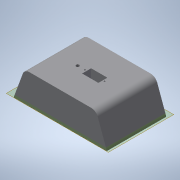
# Autodesk Inventor part: cover-new
Saved by Autodesk Inventor 2020 (Build 240168000, 168)
## iProperties
Created: 2020-08-26
Part Number: cover-new
Material: Ogólny
Document SubType Name: Modeling
Designer: blep
Density: 1 g/cm^3
Appearance: Domyślna
Author: blep
Autodesk Inventor part; units mm, degrees
ref_plane "YZ Plane" through (0, 0, 0) normal (1, 0, 0) x (0, 1, 0)
ref_plane "XZ Plane" through (0, 0, 0) normal (0, 1, 0) x (-1, 0, 0)
ref_plane "XY Plane" through (0, 0, 0) normal (0, 0, 1) x (1, 0, 0)
sketch "Szkic1" plane through (0, 0, 0) normal (0, 0, 1) x (1, 0, 0)
  line L0 (-135, 20) -> (0, 20) projected
  line L1 (-135, 7) -> (-135, 20) projected
  line L2 (0, 7) -> (0, 20) projected
  line L3 (-135, 20) -> (-119.3493, 63)
  line L4 (-119.3493, 63) -> (-15.6507, 63)
  line L5 (-15.6507, 63) -> (0, 20)
  line L6 (-135, 20) -> (-131.8075, 20)
  line L7 (-131.8075, 20) -> (-117.2487, 60)
  line L8 (-117.2487, 60) -> (-17.7513, 60)
  line L9 (-17.7513, 60) -> (-3.1925, 20)
  line L10 (-3.1925, 20) -> (0, 20)
  point P0 (0, 0)
  point P1 (-3.1925, 20)
  dimension "d0" = 3
  dimension "d1" = 3
  dimension "d2" = 3
  dimension "d3" = 40
  dimension "d4" = 70
  dimension "d5" = 70
  constraints: 16 end point, 4 horizontal, 3 parallel
  measures "d0" distance between parallel lines of L3 L7
  measures "d1" distance between parallel lines of L4 L8
  measures "d2" distance between parallel lines of L5 L9
  measures "d3" distance between parallel lines of L8 L0
  measures "d4" angle of L0 L7
  measures "d5" angle of L0 L9
ref_plane "Płaszczyzna konstrukcyjna1" through (-135, -3, -86) normal (0, 0, -1) x (0, 1, 0)
extrude "Wyciągnięcie proste1" add sketch "Szkic1" against normal up to surface (86 mm away) contours L3 L4 L5 L0 L9 L8 L7
sketch "Szkic2" plane through (0, 0, 0) normal (0, 0, 1) x (1, 0, 0)
  line L0 (-131.8075, 20) -> (-117.2487, 60) projected
  line L1 (-117.2487, 60) -> (-17.7513, 60) projected
  line L2 (-17.7513, 60) -> (-3.1925, 20) projected
  line L3 (-131.8075, 20) -> (-3.1925, 20)
  point P0 (0, 0)
  constraints: 2 end point, 1 horizontal
ref_plane "Płaszczyzna konstrukcyjna2" through (-135, -3, -86) normal (0, 0, -1) x (0, 1, 0)
extrude "Wyciągnięcie proste2" add sketch "Szkic2" against normal up to surface (86 mm away)
extrude "Wyciągnięcie proste3" cut sketch "Szkic2" against normal blind 83
extrude "Wyciągnięcie proste4" add sketch "Szkic2" against normal blind 3
sketch "Szkic3" plane through (-135, 20, -86) normal (-0.9396926, 0.3420201, 0) x (0, 0, 1)
  circle A0 centre (63.5, 28.7596) radius 7.75
  line L0 (15, 36.7596) -> (42, 36.7596)
  line L1 (42, 36.7596) -> (42, 16.7596)
  line L2 (42, 16.7596) -> (15, 16.7596)
  line L3 (15, 16.7596) -> (15, 36.7596)
  line L4 (22, 16.7596) -> (35, 16.7596)
  line L5 (35, 16.7596) -> (35, 13.7596)
  line L6 (35, 13.7596) -> (22, 13.7596)
  line L7 (22, 13.7596) -> (22, 16.7596)
  line L8 (86, 45.7596) -> (0, 45.7596) projected
  line L9 (0, 45.7596) -> (0, 0) projected
  line L10 (86, 0) -> (0, 0) projected
  line L11 (86, 45.7596) -> (86, 0) projected
  line L12 (86, 45.7596) -> (0, 45.7596) projected
  line L13 (86, 0) -> (0, 0) construction
  line L14 (42, 36.7596) -> (63.5, 28.7596) construction
  line L15 (15, 20.7596) -> (42, 20.7596) construction
  line L16 (42, 20.7596) -> (63.5, 28.7596) construction
  point P0 (86, 27.3789)
  dimension "d14" = 27
  dimension "d15" = 20
  dimension "d16" = 3
  dimension "d17" = 7
  dimension "d18" = 7
  dimension "d19" = 15.5
  dimension "d20" = 17
  dimension "d23" = 15
  dimension "d36" = 4
  dimension "d42" = 22.5
  constraints: 22 end point, 4 parallel, 3 horizontal, 2 perpendicular, 2 point on line, 1 centre point, 1 collinear, 1 equal length
  measures "d14" distance of L1.end L2.end
  measures "d15" distance of L0.end L1.end
  measures "d16" distance of L4.end L5.end
  measures "d17" distance between parallel lines of L3 L7
  measures "d18" distance between parallel lines of L1 L5
  measures "d19" diameter of A0
  measures "d20" distance from line of L8 L14.end
  measures "d23" distance between parallel lines of L9 L3
  measures "d36" distance between parallel lines of L4 L15
  measures "d42" distance from line of L11 L14.end
extrude "Wyciągnięcie proste5" cut sketch "Szkic3" against normal up to surface (3 mm away) contours A0 | L0 L1 L2 L3 | L2 L5 L6 L7
sketch "Szkic4" plane through (-135, 20, -86) normal (-0.9396926, 0.3420201, 0) x (0, 0, 1)
  line L0 (15, 20.7596) -> (42, 20.7596)
  line L1 (42, 20.7596) -> (42, 16.7596)
  line L2 (42, 16.7596) -> (15, 16.7596)
  line L3 (15, 16.7596) -> (15, 20.7596)
  line L4 (22, 16.7596) -> (35, 16.7596)
  line L5 (35, 16.7596) -> (35, 13.7596)
  line L6 (35, 13.7596) -> (22, 13.7596)
  line L7 (22, 13.7596) -> (22, 16.7596)
  line L8 (35, 13.7596) -> (22, 13.7596) projected
  line L9 (22, 13.7596) -> (22, 16.7596) projected
  line L10 (35, 16.7596) -> (35, 13.7596) projected
  line L11 (42, 36.7596) -> (42, 16.7596) projected
  line L12 (15, 16.7596) -> (15, 36.7596) projected
  line L13 (22, 16.7596) -> (15, 16.7596) projected
  point P0 (86, 27.3789)
  dimension "d26" = 4
  constraints: 16 end point, 7 collinear, 4 parallel, 2 horizontal, 2 perpendicular
  measures "d26" distance between parallel lines of L2 L0
extrude "Wyciągnięcie proste6" add sketch "Szkic4" against normal blind 1
fillet "Zaokrąglenie1" radius 10 2 edges at (-119.3493, 63, -43) (-15.6507, 63, -43)
sketch "Szkic5" plane through (0, 0, 0) normal (0, 0, 1) x (1, 0, 0)
  line L0 (-121.7441, 56.4202) -> (-135, 20) projected
  line L1 (-135, 7) -> (-135, 20) projected
  line L2 (-135, 20) -> (0, 20) projected
  arc A0 (-112.3472, 63) -> (-121.7441, 56.4202) centre (-112.3472, 53) ccw projected
  line L3 (-133.7939, 23.3139) -> (-121.7441, 56.4202)
  line L4 (-135, 16.4735) -> (-135, 7)
  arc A1 (-133.7939, 23.3139) -> (-135, 16.4735) centre (-115, 16.4735) ccw
  line L5 (0, 7) -> (0, 20) projected
  line L6 (0, 20) -> (-13.2559, 56.4202) projected
  line L7 (0, 16.4735) -> (0, 7)
  line L8 (0, 20) -> (-13.2559, 56.4202) projected
  line L9 (-1.2061, 23.3139) -> (-13.2559, 56.4202)
  arc A2 (0, 16.4735) -> (-1.2061, 23.3139) centre (-20, 16.4735) ccw
  line L10 (0, 7) -> (-135, 7)
  line L11 (-121.7441, 56.4202) -> (-119.3493, 63)
  line L12 (-119.3493, 63) -> (-15.6507, 63)
  line L13 (-15.6507, 63) -> (-13.2559, 56.4202)
  line L14 (-22.6528, 63) -> (-112.3472, 63) projected
  point P0 (0, 0)
  dimension "d30" = 20
  dimension "d31" = 20
  constraints: 16 end point, 6 collinear, 5 tangent, 4 point on circle, 4 point on line, 2 centre point, 1 perpendicular, 1 vertical
  measures "d30" radius of A1
  measures "d31" radius of A2
extrude "Wyciągnięcie proste7" cut sketch "Szkic5" against normal through all contours A0 L12 L13 L6 A2 L2 A1 L0 | L2 A2 L5 L10 L1 A1 keep common part
sketch "Szkic6" plane through (-134.6866, 20, 0) normal (0, -1, 0) x (1, 0, 0)
  arc A0 (2.8554, -3) -> (2.6866, -3.1688) centre (5.6866, -6) ccw projected
  line L0 (2.8554, -3) -> (2.6866, -3) projected
  line L1 (2.6866, -3) -> (2.6866, -3.1688) projected
  circle A1 centre (128.6866, -6) radius 2.125 projected
  circle A2 centre (128.6866, -80) radius 2.125 projected
  circle A3 centre (5.6866, -80) radius 2.125 projected
  line L2 (2.6866, -82.8312) -> (2.6866, -83) projected
  line L3 (2.6866, -83) -> (2.8554, -83) projected
  arc A4 (2.6866, -82.8312) -> (2.8554, -83) centre (5.6866, -80) ccw projected
  circle A5 centre (5.6866, -6) radius 2.125 projected
  line L4 (2.6866, -8.8312) -> (2.6866, -77.1688) projected
  arc A6 (8.5178, -83) -> (2.6866, -77.1688) centre (5.6866, -80) ccw projected
  line L5 (8.5178, -83) -> (71.1366, -83) projected
  line L6 (71.1366, -83) -> (71.1366, -75.35) projected
  line L7 (71.1366, -75.35) -> (79.1366, -75.35) projected
  line L8 (79.1366, -75.35) -> (79.1366, -83) projected
  line L9 (79.1366, -83) -> (120.2366, -83) projected
  line L10 (120.2366, -83) -> (120.2366, -75.35) projected
  line L11 (120.2366, -75.35) -> (131.6866, -75.35) projected
  line L12 (131.6866, -75.35) -> (131.6866, -10.65) projected
  line L13 (131.6866, -10.65) -> (120.2366, -10.65) projected
  line L14 (120.2366, -10.65) -> (120.2366, -3) projected
  line L15 (120.2366, -3) -> (79.1366, -3) projected
  line L16 (79.1366, -3) -> (79.1366, -10.65) projected
  line L17 (79.1366, -10.65) -> (71.1366, -10.65) projected
  line L18 (71.1366, -10.65) -> (71.1366, -3) projected
  line L19 (71.1366, -3) -> (8.5178, -3) projected
  arc A7 (2.6866, -8.8312) -> (8.5178, -3) centre (5.6866, -6) ccw projected
  line L20 (0, 0) -> (0, -86) projected
  line L21 (0, 0) -> (134.3733, 0) projected
  line L22 (134.3733, -86) -> (134.3733, 0) projected
  line L23 (134.3733, -86) -> (0, -86) projected
  circle A8 centre (5.6866, -6) radius 4.125
  circle A9 centre (5.6866, -6) radius 2.125
  circle A10 centre (128.6866, -6) radius 2.125
  circle A11 centre (128.6866, -6) radius 4.125
  circle A12 centre (128.6866, -80) radius 2.125
  circle A13 centre (128.6866, -80) radius 4.125
  circle A14 centre (5.6866, -80) radius 2.125
  circle A15 centre (5.6866, -80) radius 4.125
  point P0 (134.6866, 0)
  point P1 (2.6866, -3.1688)
  point P2 (2.8554, -3)
  point P3 (8.5178, -83)
  point P4 (2.6866, -77.1688)
  constraints: 8 centre point, 8 coincident, 8 equal radius
extrude "Wyciągnięcie proste8" add sketch "Szkic6" against normal through all contours A8 A7 A0 | A6 A15 A4 | A11 | A13
ref_plane "Płaszczyzna konstrukcyjna3" through (-134.6866, 24, 0) normal (0, -1, 0) x (1, 0, 0)
sketch "Szkic11" plane through (-134.6866, 24, 0) normal (0, -1, 0) x (1, 0, 0)
  arc A0 (8.5178, -83) -> (2.8792, -76.9778) centre (5.6866, -80) ccw projected
  arc A1 (125.8554, -3) -> (131.4941, -9.0222) centre (128.6866, -6) ccw projected
  arc A2 (131.4941, -76.9778) -> (125.8554, -83) centre (128.6866, -80) ccw projected
  arc A3 (2.8792, -9.0222) -> (8.5178, -3) centre (5.6866, -6) ccw projected
  circle A4 centre (5.6866, -80) radius 4.125
  circle A5 centre (5.6866, -6) radius 4.125
  circle A6 centre (128.6866, -6) radius 4.125
  circle A7 centre (128.6866, -80) radius 4.125
  circle A8 centre (128.6866, -80) radius 2.125 projected
  circle A9 centre (128.6866, -6) radius 2.125 projected
  circle A10 centre (5.6866, -80) radius 2.125 projected
  circle A11 centre (5.6866, -6) radius 2.125 projected
  point P0 (8.5178, -3)
  point P1 (131.4941, -9.0222)
  point P2 (125.8554, -3)
  point P3 (125.8554, -83)
  point P4 (2.8792, -76.9778)
  constraints: 4 centre point, 4 coincident, 4 concentric
extrude "Wyciągnięcie proste9" cut sketch "Szkic11" along normal blind 3 contours A4 A0 | A6 A1 | A7 A2 | A5 A3 | A8 | A9 | A10 | A11
sketch "Szkic12" plane through (-134.6866, 20, 0) normal (0, -1, 0) x (1, 0, 0)
  circle A0 centre (5.6866, -80) radius 2.125 projected
  circle A1 centre (128.6866, -6) radius 2.125 projected
  line L0 (134.3733, 0) -> (134.3733, -86) projected
  line L1 (0, 0) -> (134.3733, 0) projected
  line L2 (0, -86) -> (0, 0) projected
  line L3 (0, -86) -> (134.3733, -86) projected
  circle A2 centre (5.6866, -6) radius 2.125 projected
  circle A3 centre (128.6866, -80) radius 2.125 projected
  arc A4 (131.4941, -76.9778) -> (125.8554, -83) centre (128.6866, -80) ccw projected
  line L4 (125.8554, -83) -> (8.5178, -83) projected
  arc A5 (8.5178, -83) -> (2.8792, -76.9778) centre (5.6866, -80) ccw projected
  line L5 (2.8792, -76.9778) -> (2.8792, -9.0222) projected
  arc A6 (2.8792, -9.0222) -> (8.5178, -3) centre (5.6866, -6) ccw projected
  line L6 (125.8554, -3) -> (8.5178, -3) projected
  arc A7 (125.8554, -3) -> (131.4941, -9.0222) centre (128.6866, -6) ccw projected
  line L7 (131.4941, -9.0222) -> (131.4941, -76.9778) projected
  point P0 (134.6866, 0)
extrude "Wyciągnięcie proste10" cut sketch "Szkic12" against normal blind 8 contours A0 | A1 | A2 | A3
sketch "Szkic13" plane through (-112.3472, 63, -86) normal (0, 1, 0) x (1, 0, 0)
  line L0 (68.5, -49.5) -> (35, -49.5)
  line L1 (35, -49.5) -> (35, -36.5)
  line L2 (35, -36.5) -> (68.5, -36.5)
  line L3 (68.5, -36.5) -> (68.5, -49.5)
  line L4 (89.6944, -86) -> (0, -86) projected
  line L5 (89.6944, 0) -> (0, 0) projected
  line L6 (89.6944, 0) -> (89.6944, -86) projected
  line L7 (0, -86) -> (0, 0) projected
  line L8 (99.0913, -86) -> (89.6944, -86) construction
  line L9 (68.5, -49.5) -> (89.6944, -86) construction
  line L10 (68.5, -36.5) -> (89.6944, 0) construction
  line L11 (63.5, -49.5) -> (63.5, -36.5)
  line L12 (40, -49.5) -> (40, -36.5)
  line L13 (68.5, -49.5) -> (66, -43) construction
  line L14 (66, -43) -> (63.5, -36.5) construction
  line L15 (68.5, -36.5) -> (66, -43) construction
  line L16 (40, -49.5) -> (37.5, -43) construction
  line L17 (37.5, -43) -> (35, -36.5) construction
  line L18 (37.5, -43) -> (40, -36.5) construction
  circle A0 centre (27, -43) radius 2.25
  line L19 (0, -86) -> (27, -43) construction
  line L20 (0, 0) -> (27, -43) construction
  circle A1 centre (57, -43) radius 1.5065 construction
  point P0 (112.3472, -86)
  dimension "d70" = 13
  dimension "d71" = 33.5
  dimension "d72" = 5
  dimension "d73" = 5
  dimension "d86" = 35
  dimension "d87" = 4.5
  dimension "d88" = 30
  constraints: 32 end point, 6 equal length, 4 parallel, 4 point on line, 2 centre point, 1 horizontal, 1 perpendicular, 2 other
  measures "d70" distance of L0.end L1.end
  measures "d71" distance of L1.end L2.end
  measures "d72" distance between parallel lines of L3 L11
  measures "d73" distance between parallel lines of L1 L12
  measures "d86" distance between parallel lines of L7 L1
  measures "d87" diameter of A0
  measures "d88" distance of L19.end A1.centre
extrude "Wyciągnięcie proste11" cut sketch "Szkic13" against normal through all contours L0 L12 L2 L11
hole "Otwór1" at (-46.3472, 63, -43) at (-74.8472, 63, -43) direction (0, -1, 0) diameter 2 end through all
sketch "Szkic14" plane through (-117.2487, 60, -83) normal (0, -1, 0) x (1, 0, 0)
  circle A0 centre (70.9015, 40) radius 1 projected
  circle A1 centre (42.4015, 40) radius 1 projected
  line L0 (68.4015, 46.5) -> (68.4015, 33.5) projected
  line L1 (68.4015, 33.5) -> (44.9015, 33.5) projected
  line L2 (44.9015, 33.5) -> (44.9015, 46.5) projected
  line L3 (44.9015, 46.5) -> (68.4015, 46.5) projected
  line L4 (99.4973, 80) -> (0, 80) projected
  line L5 (0, 80) -> (0, 0) projected
  line L6 (0, 0) -> (99.4973, 0) projected
  line L7 (99.4973, 80) -> (99.4973, 0) projected
  line L8 (42.9015, 31.5) -> (70.4015, 31.5)
  line L9 (70.4015, 31.5) -> (70.4015, 48.5)
  line L10 (70.4015, 48.5) -> (42.9015, 48.5)
  line L11 (42.9015, 48.5) -> (42.9015, 31.5)
  point P0 (117.2487, 83)
  point P1 (42.9015, 40.866)
  point P2 (42.9015, 39.134)
  point P3 (70.4015, 39.134)
  point P4 (70.4015, 40.866)
  dimension "d83" = 2
  constraints: 8 end point, 3 other
  measures "d83" distance between parallel lines of L1 L8
extrude "Wyciągnięcie proste12" add sketch "Szkic14" along normal blind 10 contours A0 L9 L8 L11 A1 L10
extrude "Wyciągnięcie proste13" cut sketch "Szkic13" against normal through all contours A0
equation "\"d1\" = d0"
equation "\"d2\" = d0"
equation "\"d5\" = d4"
equation "\"d18\" = d17"
equation "\"d31\" = d30"
equation "\"d73\" = d72"
